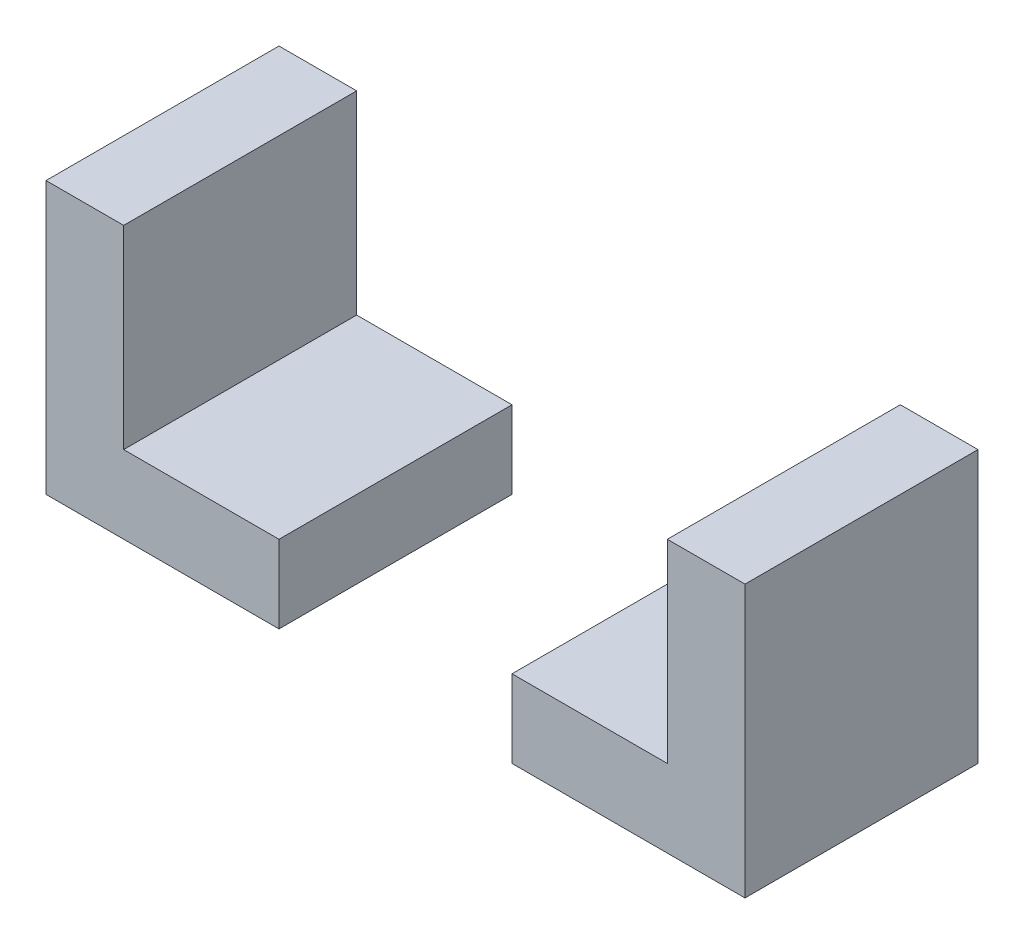
# Autodesk Inventor part: Guide_Basic
Saved by Autodesk Inventor 2026.1 (Build 301233020, 233B)
## iProperties
Created: 2026-03-11
Part Number: Guide_Basic
Material: Generic
Document SubType Name: Modeling
Designer: elaij
Density: 1 g/cm^3
Appearance: Default
Author: elaij
Autodesk Inventor part; units mm, degrees
ref_plane "YZ Plane" through (0, 0, 0) normal (1, 0, 0) x (0, 1, 0)
ref_plane "XZ Plane" through (0, 0, 0) normal (0, 1, 0) x (-1, 0, 0)
ref_plane "XY Plane" through (0, 0, 0) normal (0, 0, 1) x (1, 0, 0)
sketch "Sketch2" plane through (0, 0, 0) normal (0, 0, 1) x (1, 0, 0)
  line L0 (15, 0) -> (35, 0)
  line L1 (35, 0) -> (35, 10)
  line L2 (35, 10) -> (15, 10)
  line L3 (15, 10) -> (15, 0)
  line L4 (35, 0) -> (45, 0)
  line L5 (45, 0) -> (45, 35)
  line L6 (45, 35) -> (35, 35)
  line L7 (35, 35) -> (35, 0)
  line L8 (0, 0) -> (0, 15.6723)
  line L9 (-15, 0) -> (-35, 0)
  line L10 (-35, 0) -> (-35, 10)
  line L11 (-35, 10) -> (-15, 10)
  line L12 (-15, 10) -> (-15, 0)
  line L13 (-35, 0) -> (-45, 0)
  line L14 (-45, 0) -> (-45, 35)
  line L15 (-45, 35) -> (-35, 35)
  line L16 (-35, 35) -> (-35, 0)
  point P0 (35, 10)
  point P1 (-35, 10)
  dimension "d15" = 15
  dimension "d16" = 10
  dimension "d17" = 20
  dimension "d18" = 10
  dimension "d19" = 35
  dimension "d20" = 35
  constraints: 34 end point, 7 symmetric about line, 4 parallel, 2 horizontal, 2 perpendicular, 1 vertical
  measures "d15" distance from line of L8.start L3
  measures "d16" distance between parallel lines of L0 L2
  measures "d17" distance between parallel lines of L1 L3
  measures "d18" distance between parallel lines of L5 L7
  measures "d19" distance between parallel lines of L4 L6
  measures "d20" distance from line of L8.start L6
extrude "Extrusion2" add sketch "Sketch2" along normal blind 30
body "Solid2"
